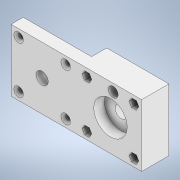
# Autodesk Inventor part: ReductionGearBracket
Saved by Autodesk Inventor 2021 (Build 250183000, 183)
## iProperties
Created: 2020-08-25
Part Number: ReductionGearBracket
Material: Generic
Document SubType Name: Modeling
Designer: elmar
Density: 1 g/cm^3
Appearance: White
Author: elmar
Autodesk Inventor part; units mm, degrees
ref_plane "YZ Plane" through (0, 0, 0) normal (1, 0, 0) x (0, 1, 0)
ref_plane "XZ Plane" through (0, 0, 0) normal (0, 1, 0) x (-1, 0, 0)
ref_plane "XY Plane" through (0, 0, 0) normal (0, 0, 1) x (1, 0, 0)
sketch "Sketch1" plane through (0, 0, 0) normal (0, 0, 1) x (1, 0, 0)
  line L0 (-15.5, 15.5) -> (15.5, 15.5)
  line L1 (15.5, 15.5) -> (15.5, -15.5)
  line L2 (15.5, -15.5) -> (-15.5, -15.5)
  line L3 (-15.5, -15.5) -> (-15.5, 15.5)
  line L4 (29.5, 15.5) -> (60.5, 15.5)
  line L5 (60.5, 15.5) -> (60.5, -15.5)
  line L6 (60.5, -15.5) -> (29.5, -15.5)
  line L7 (29.5, -15.5) -> (29.5, 15.5)
  line L8 (-20.5, 20.5) -> (65.5, 20.5)
  line L9 (65.5, 20.5) -> (65.5, -20.5)
  line L10 (65.5, -20.5) -> (-20.5, -20.5)
  line L11 (-20.5, -20.5) -> (-20.5, 20.5)
  circle A0 centre (0, 0) radius 11
  circle A1 centre (45, 0) radius 11
  dimension "d0" = 31
  dimension "d5" = 45
  dimension "d10" = 5
  dimension "d11" = 5
  dimension "d12" = 5
  dimension "d13" = 5
  dimension "d16" = 22
  constraints: 24 end point, 3 coincident, 2 centre point, 2 horizontal, 2 parallel, 1 collinear, 1 equal radius, 1 perpendicular, 1 vertical, 17 other
  measures "d0" distance of L0.start L0.end
  measures "d5" distance of point (0, 0) point (45, 0)
  measures "d10" distance between parallel lines of L8 L0
  measures "d11" distance between parallel lines of L11 L3
  measures "d12" distance between parallel lines of L10 L2
  measures "d13" distance between parallel lines of L5 L9
  measures "d16" diameter of A0
extrude "Extrusion1" add sketch "Sketch1" along normal blind 8 contours L0 L1 L2 L3 | L4 L5 L6 L7 | L8 L9 L10 L11 | A0 | A1
sketch "Sketch2" plane through (0, 0, 0) normal (0, 0, 1) x (1, 0, 0)
  circle A0 centre (45, 0) radius 11 projected
  point P0 (0, 0)
sketch "Sketch4" plane through (0, 0, 8) normal (0, 0, 1) x (1, 0, 0)
  point P0 (0, 0)
  point P1 (15.5, 15.5)
  point P2 (-15.5, 15.5)
  point P3 (-15.5, -15.5)
  point P4 (15.5, -15.5)
hole "Hole3" at (-15.5, 15.5, 8) at (15.5, 15.5, 8) at (15.5, -15.5, 8) at (-15.5, -15.5, 8) direction (0, 0, -1) diameter 3.2 end through all countersink diameter 6.3 countersink angle 90 clearance for "Flat Head Machine Screw" size "M3" standard "Ansi Metric M Profile"
sketch "Sketch16" plane through (0, 0, 0) normal (0, 0, 1) x (1, 0, 0)
  line L0 (65.5, 20.5) -> (-20.5, 20.5) projected
  line L1 (-20.5, -20.5) -> (65.5, -20.5) projected
  line L2 (24.5, 20.5) -> (65.5, 20.5)
  line L3 (65.5, 20.5) -> (65.5, -20.5)
  line L4 (65.5, -20.5) -> (24.5, -20.5)
  line L5 (24.5, -20.5) -> (24.5, 20.5)
  point P0 (0, 0)
  constraints: 8 end point, 2 parallel, 2 perpendicular, 1 horizontal, 1 point on line
extrude "Extrusion7" add sketch "Sketch16" against normal blind 10
sketch "Sketch18" plane through (0, 0, 8) normal (0, 0, 1) x (1, 0, 0)
  line L0 (29.5, 15.5) -> (60.5, 15.5) projected
  line L1 (29.5, -15.5) -> (29.5, 15.5) projected
  line L2 (60.5, -15.5) -> (29.5, -15.5) projected
  line L3 (60.5, 15.5) -> (60.5, -15.5) projected
  point P0 (0, 0)
sketch "Sketch14" plane through (0, 0, 8) normal (0, 0, -1) x (-1, 0, 0)
  circle A0 centre (-45, 0) radius 11 projected
  point P0 (0, 0)
  point P1 (-46.783, 15.548)
  dimension "d178" = 1.783
  dimension "d179" = 15.548
  measures "d178" horizontal distance of point (-46.783, 15.548) A0.centre
  measures "d179" vertical distance of point (-46.783, 15.548) A0.centre
hole "Hole5" at (46.783, 15.548, 8) direction (0, 0, -1) diameter 6.5 end through all
sketch "Sketch13" plane through (0, 0, 8) normal (0, 0, -1) x (-1, 0, 0)
  line L0 (-62.0877, 18.25) -> (-58.9123, 18.25)
  line L1 (-58.9123, 18.25) -> (-57.3246, 15.5)
  line L2 (-57.3246, 15.5) -> (-58.9123, 12.75)
  line L3 (-58.9123, 12.75) -> (-62.0877, 12.75)
  line L4 (-62.0877, 12.75) -> (-63.6754, 15.5)
  line L5 (-63.6754, 15.5) -> (-62.0877, 18.25)
  line L6 (-31.0877, 18.25) -> (-27.9123, 18.25)
  line L7 (-27.9123, 18.25) -> (-26.3246, 15.5)
  line L8 (-26.3246, 15.5) -> (-27.9123, 12.75)
  line L9 (-27.9123, 12.75) -> (-31.0877, 12.75)
  line L10 (-31.0877, 12.75) -> (-32.6754, 15.5)
  line L11 (-32.6754, 15.5) -> (-31.0877, 18.25)
  line L12 (-62.0877, -12.75) -> (-58.9123, -12.75)
  line L13 (-58.9123, -12.75) -> (-57.3246, -15.5)
  line L14 (-57.3246, -15.5) -> (-58.9123, -18.25)
  line L15 (-58.9123, -18.25) -> (-62.0877, -18.25)
  line L16 (-62.0877, -18.25) -> (-63.6754, -15.5)
  line L17 (-63.6754, -15.5) -> (-62.0877, -12.75)
  line L18 (-31.0877, -12.75) -> (-27.9123, -12.75)
  line L19 (-27.9123, -12.75) -> (-26.3246, -15.5)
  line L20 (-26.3246, -15.5) -> (-27.9123, -18.25)
  line L21 (-27.9123, -18.25) -> (-31.0877, -18.25)
  line L22 (-31.0877, -18.25) -> (-32.6754, -15.5)
  line L23 (-32.6754, -15.5) -> (-31.0877, -12.75)
  point P0 (0, 0)
  point P1 (-60.5, 15.5)
  point P2 (-29.5, 15.5)
  point P3 (-60.5, -15.5)
  point P4 (-29.5, -15.5)
  point P5 (-60.5, 15.5)
  point P6 (-29.5, 15.5)
  point P7 (-60.5, -15.5)
  point P8 (-29.5, -15.5)
  point P9 (-45, 0)
  dimension "d129" = 5.5
  constraints: 48 end point, 4 coincident, 4 horizontal, 2 equal length, 1 point on line, 52 other
  measures "d129" distance between parallel lines of L3 L0
extrude "Extrusion6" cut sketch "Sketch13" along normal blind 3.6
hole "Hole7" at (45, 0, 8) direction (0, 0, -1) diameter 8 end through all counterbore diameter 22 counterbore depth 7
hole "Hole8" at (29.5, 15.5, 8) at (60.5, 15.5, 8) at (60.5, -15.5, 8) at (29.5, -15.5, 8) direction (0, 0, -1) diameter 3.2 end through all clearance for "Flat Head Machine Screw" size "M3" standard "Ansi Metric M Profile"
hole "Hole9" at (0, 0, 0) direction (0, 0, 1) diameter 8 end through all counterbore diameter 23 counterbore depth 2.2
equation "\"d64\" = 55deg"
equation "\"Sketch5_Pitch\" = 0.5"
equation "\"d82\" = 55deg"
equation "\"Sketch7_Pitch\" = 0.5"
equation "\"d100\" = 55deg"
equation "\"Sketch9_Pitch\" = 0.5"
equation "\"d118\" = 55deg"
equation "\"Sketch11_Pitch\" = 0.5"
body "Solid1"
